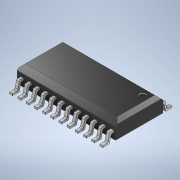
# Autodesk Inventor part: Part2
Saved by Autodesk Inventor 2021 (Build 250183000, 183)
## iProperties
Created: 2023-04-01
Part Number: Part2
Material: Generic
Document SubType Name: Modeling
Designer: stepa
Density: 1 g/cm^3
Appearance: Default
Author: stepa
Autodesk Inventor part; units mm, degrees
ref_plane "YZ Plane" through (0, 0, 0) normal (1, 0, 0) x (0, 1, 0)
ref_plane "XZ Plane" through (0, 0, 0) normal (0, 1, 0) x (-1, 0, 0)
sketch "Sketch1" plane through (0, 0, 0) normal (0, 1, 0) x (-1, 0, 0)
  line L0 (7.5, 3.6) -> (-7.5, 3.6)
  line L1 (-7.5, 3.6) -> (-7.5, -3.6)
  line L2 (-7.5, -3.6) -> (7.5, -3.6)
  line L3 (7.5, -3.6) -> (7.5, 3.6)
  line L4 (7.5, 3.6) -> (-7.5, -3.6) construction
  line L5 (-7.5, 3.6) -> (7.5, -3.6) construction
  point P0 (0, 0)
  dimension "d0" = 7.2
  dimension "d1" = 15
  constraints: 12 end point, 2 midpoint, 2 parallel, 1 horizontal, 1 perpendicular
  measures "d0" distance of L2.end L0.start
  measures "d1" distance of L1.end L2.end
extrude "Extrusion1" add sketch "Sketch1" along normal blind 2.8
ref_plane "Work Plane1" through (7, 0, 3.6) normal (1, 0, 0) x (0, 0, -1)
sketch "Sketch2" plane through (7, 0, 3.6) normal (1, 0, 0) x (0, 0, -1)
  line L0 (7.2, 0) -> (7.2, 2.8) projected
  line L1 (7.2, 1.511) -> (7.6692, 1.511)
  line L2 (7.8644, 1.3547) -> (8.0657, 0.4563)
  line L3 (8.2609, 0.3) -> (8.85, 0.3)
  line L4 (8.9, 0.25) -> (8.9, 0.05)
  line L5 (8.85, 0) -> (8.0207, 0)
  line L6 (7.8255, 0.1563) -> (7.6242, 1.0547)
  line L7 (7.429, 1.211) -> (7.2, 1.211)
  arc A0 (7.8644, 1.3547) -> (7.6692, 1.511) centre (7.6692, 1.311) ccw
  arc A1 (8.0657, 0.4563) -> (8.2609, 0.3) centre (8.2609, 0.5) ccw
  arc A2 (7.8255, 0.1563) -> (8.0207, 0) centre (8.0207, 0.2) ccw
  arc A3 (7.6242, 1.0547) -> (7.429, 1.211) centre (7.429, 1.011) ccw
  arc A4 (8.9, 0.25) -> (8.85, 0.3) centre (8.85, 0.25) ccw
  arc A5 (8.85, 0) -> (8.9, 0.05) centre (8.85, 0.05) ccw
  point P0 (3.6, 0)
  point P1 (7.8293, 1.511)
  point P2 (8.1008, 0.3)
  point P3 (8.9, 0.3)
  point P4 (8.9, 0)
  point P5 (7.8606, 0)
  point P6 (7.5891, 1.211)
  dimension "d5" = 1.7
  dimension "d6" = 0.3
  dimension "d7" = 0.3
  dimension "d8" = 0.3
  dimension "d26" = 0.2
  dimension "d27" = 0.05
  constraints: 14 end point, 14 point on line, 12 point on circle, 12 tangent, 6 centre point, 4 equal radius, 3 parallel, 3 perpendicular, 1 horizontal, 1 horizontal alignment
  measures "d5" distance between parallel lines of L4 L0
  measures "d6" distance between parallel lines of L6 L2
  measures "d7" distance between parallel lines of L5 L3
  measures "d8" distance between parallel lines of L1 L7
  measures "d26" radius of A0
  measures "d27" radius of A4
extrude "Extrusion2" add sketch "Sketch2" along normal mid plane 0.5
fillet "Fillet3" radius 0.05 26 edges at (7.25, 1.4671, -4.1942) (7.25, 1.511, -3.8346) (7.25, 0.3439, -4.5359) (7.25, 0.3, -4.9554) (7.25, 0.2854, -5.2854) (7.25, 0.15, -5.3) (7.25, 0.0146, -5.2854) (7.25, 0, -4.8353) (7.25, 0.0439, -4.2957) (7.25, 0.6055, -4.1248) (7.25, 1.1671, -3.954) (7.25, 1.211, -3.7145) (7.25, 0.9055, -4.365) (6.75, 0.3439, -4.5359) (6.75, 0.3, -4.9554) (6.75, 0.2854, -5.2854) (6.75, 0.15, -5.3) (6.75, 0.0146, -5.2854) (6.75, 0, -4.8353) (6.75, 0.0439, -4.2957) (6.75, 0.6055, -4.1248) (6.75, 1.1671, -3.954) (6.75, 1.211, -3.7145) (6.75, 1.4671, -4.1942) (6.75, 1.511, -3.8346) (6.75, 0.9055, -4.365)
chamfer "Chamfer4" distance 0.75 angle 45 2 edges at (0, 2.8, -3.6) (0, 2.8, 3.6)
chamfer "Chamfer5" distance 0.5 angle 45 2 edges at (7.5, 2.8, 0) (-7.5, 2.8, 0)
chamfer "Chamfer6" distance 0.3 angle 45 4 edges at (7.5, 0, 0) (0, 0, 3.6) (0, 0, -3.6) (-7.5, 0, 0)
pattern_linear "Rectangular Pattern2" count 12 spacing 1.25 along (-1, 0, 0) of "Fillet3", "Extrusion2"
mirror "Mirror2" about plane through (0, 0, 0) normal (0, 0, 1) of "Fillet3", "Extrusion2", "Rectangular Pattern2"
sketch "Sketch4" plane through (0, 2.8, 0) normal (0, 1, 0) x (1, 0, 0)
  circle A0 centre (6.0998, 1.9324) radius 0.4785
  point P0 (0, 0)
  constraints: 1 centre point
extrude "Extrusion4" cut sketch "Sketch4" against normal blind 0.2
body "Solid1"
